Autodesk Fusion 360 part; units mm, degrees
note: some values were not read from the file. Chosen so that the rebuilt part matches the saved one: which bodies a step acts on; a direction; that a step has no effect; which face or edge a step refers to; which pieces of a blend or face edit are solid. Set by a fixed rule: which sketch regions a step uses.
(part 2 of 3)
sketch "Skizze17" plane through (0, 0, -29.4) normal (0, 0, 1) x (1, 0, 0)
  line L0 (185, -2.4) -> (185, 0)
  line L1 (-9.4, 0) -> (-9.4, -2.4)
  line L2 (77.8, 90) -> (97.8, 90)
  line L3 (97.8, 90) -> (97.8, 105)
  line L4 (97.8, 105) -> (77.8, 105)
  line L5 (77.8, 105) -> (77.8, 90)
  circle A0 centre (87.8, 99) radius 2.05
  line L6 (185, -2.4) -> (185, 0)
  line L7 (185, 0) -> (185, 90)
  line L8 (10.6, 105) -> (10.6, 90)
  line L9 (30.6, 90) -> (30.6, 105)
  circle A1 centre (20.6, 99) radius 2.05
  line L10 (10.6, 90) -> (30.6, 90)
  line L11 (30.6, 105) -> (10.6, 105)
  line L12 (185, 0) -> (-9.4, 0)
  line L13 (-9.4, -2.4) -> (185, -2.4)
  dimension "d286" = 20
  dimension "d290" = 4.1
  dimension "d291" = 10
  dimension "d693" = 20
  dimension "d694" = 4.1
  dimension "d695" = 10
  dimension "d701" = 20
  dimension "d703" = 97.2
  dimension "d704" = 99.3749
  dimension "d705" = 15
  dimension "d710" = 6
  constraint horizontal L2
  constraint vertical L3
  constraint horizontal L4
  constraint vertical L5
  constraint horizontal L10
  constraint vertical L9
  constraint horizontal L11
  constraint vertical L8
  constraint horizontal L4.end L9.end
  constraint horizontal A0.centre A1.centre
  measures "d286" distance of L2.start L2.end
  measures "d290" diameter of A0
  measures "d291" distance of L3 A0.centre
  measures "d693" distance of L8.end L9.start
  measures "d694" diameter of A1
  measures "d695" distance of A1.centre L9
  measures "d701" distance of L1.start L8
  measures "d703" distance of L1 A0.centre
  measures "d705" distance of L10 L11
  measures "d710" distance of A1.centre L11
extrude "Extrusion27" add sketch "Skizze17" along normal blind 2.4 from surface at -130.8 contours L2 L3 L4 L5 | L8 L9 L10 L11 bodies 5
sketch "Skizze18" plane through (-9.4, 0, 0) normal (-1, 0, 0) x (0, 0, 1)
  line L0 (8.8, 0) -> (8.8, 81.8)
  line L1 (-120.2, 90) -> (-120.2, 105)
  line L2 (-120.2, 105) -> (-140.2, 105)
  line L3 (-140.2, 105) -> (-140.2, 90)
  circle A0 centre (-130.2, 99) radius 2.05
  line L4 (-29.4, -2.4) -> (-29.4, 0)
  line L5 (-160.2, -2.4) -> (-29.4, -2.4)
  line L6 (-140.2, 90) -> (-120.2, 90)
  line L7 (-49.4, 105) -> (-69.4, 105)
  line L8 (-69.4, 90) -> (-49.4, 90)
  line L9 (-69.4, 105) -> (-69.4, 90)
  line L10 (-49.4, 90) -> (-49.4, 105)
  circle A1 centre (-59.4, 99) radius 2.05
  line L11 (-29.4, 0) -> (-29.4, 90)
  line L12 (-160.2, 90) -> (-29.4, 90)
  line L13 (-29.4, 90) -> (-160.2, 90)
  line L14 (-160.2, 0) -> (-160.2, -2.4)
  line L15 (-29.4, 0) -> (-160.2, 0)
  line L16 (-160.2, 0) -> (-29.4, 0)
  line L17 (-29.4, 0) -> (-29.4, 90)
  line L18 (-160.2, 90) -> (-160.2, 0)
  point P0 (-160.2, 90)
  dimension "d298" = 20
  dimension "d299" = 15
  dimension "d300" = 4.1
  dimension "d301" = 10
  dimension "d687" = 20
  dimension "d688" = 15
  dimension "d689" = 4.1
  dimension "d690" = 10
  dimension "d692" = 20
  dimension "d707" = 6
  dimension "d708" = 6
  dimension "d709" = 20
  constraint vertical L1
  constraint horizontal L2
  constraint vertical L3
  constraint coincident L1 L6.end
  constraint perpendicular L1 L6
  constraint vertical L10
  constraint horizontal L7
  constraint vertical L9
  constraint coincident L8.end L10
  constraint perpendicular L8 L10
  constraint coincident L3.end L12
  constraint coincident L8.start L12
  measures "d298" distance of L3.end L1.start
  measures "d299" distance of L3.end L2.end
  measures "d300" diameter of A0
  measures "d301" distance of L1 A0.centre
  measures "d687" distance of L8.end L8.start
  measures "d688" distance of L8.start L7.end
  measures "d689" diameter of A1
  measures "d690" distance of A1.centre L10
  measures "d692" distance of L10 L11
  measures "d707" distance of A1.centre L7
  measures "d708" distance of L2 A0.centre
  measures "d709" distance of L3 P0
extrude "Extrusion28" add sketch "Skizze18" against normal up to surface (2.4 mm away) contours L1 L2 L3 L6 L12 L13 | L7 L8 L9 L10 L12 L13 bodies 5
chamfer "Fase10" distance 6 distance2 7 4 edges at (97.8, 105, -159) (30.6, 105, -159) (-8.2, 105, -120.2) (-8.2, 105, -49.4) measured on face at (97.8, 95, -158.6) measured on face at (30.6, 95, -158.6) measured on face at (-8.6, 105, -126.8667) measured on face at (-7.8, 105, -56.0667) on bodies 5
chamfer "Fase11" distance 7 distance2 6 4 edges at (-8.2, 105, -69.4) (-8.2, 105, -140.2) (10.6, 105, -159) (77.8, 105, -159) measured on face at (-8.6, 100, -69.4) measured on face at (-8.6, 100, -140.2) measured on face at (14.9333, 105, -159.4) measured on face at (86.4667, 105, -158.6) on bodies 5
sketch "Skizze11" plane through (0, 0, 0) normal (0, 1, 0) x (1, 0, 0)
  line L0 (142.6, 34.4) -> (22.6, 34.4)
  line L1 (22.6, 34.4) -> (22.6, 154.4)
  line L2 (22.6, 154.4) -> (142.6, 154.4)
  line L3 (142.6, 154.4) -> (142.6, 34.4)
  circle A0 centre (82.6, 94.4) radius 57.5
  circle A1 centre (29.6, 147.4) radius 2.5
  circle A2 centre (29.6, 41.4) radius 2.5
  circle A3 centre (135.6, 41.4) radius 2.5
  circle A4 centre (135.6, 147.4) radius 2.5
  line L4 (185, 29.4) -> (185, 160.2)
  circle A5 centre (29.6, 147.4) radius 1.375
  circle A6 centre (135.6, 147.4) radius 1.375
  circle A7 centre (135.6, 41.4) radius 1.375
  circle A8 centre (29.6, 41.4) radius 1.375
  line L5 (22.6, 146.4) -> (142.6, 146.4)
  line L6 (142.6, 146.4) -> (142.6, 142.4)
  line L7 (142.6, 142.4) -> (22.6, 142.4)
  line L8 (22.6, 142.4) -> (22.6, 146.4)
  line L9 (142.6, 140.4) -> (22.6, 140.4)
  line L10 (22.6, 140.4) -> (22.6, 136.4)
  line L11 (22.6, 136.4) -> (142.6, 136.4)
  line L12 (142.6, 136.4) -> (142.6, 140.4)
  line L13 (22.6, 134.4) -> (142.6, 134.4)
  line L14 (142.6, 134.4) -> (142.6, 130.4)
  line L15 (142.6, 130.4) -> (22.6, 130.4)
  line L16 (22.6, 130.4) -> (22.6, 134.4)
  line L17 (142.6, 128.4) -> (22.6, 128.4)
  line L18 (22.6, 128.4) -> (22.6, 124.4)
  line L19 (22.6, 124.4) -> (142.6, 124.4)
  line L20 (142.6, 124.4) -> (142.6, 128.4)
  line L21 (22.6, 122.4) -> (142.6, 122.4)
  line L22 (142.6, 122.4) -> (142.6, 118.4)
  line L23 (142.6, 118.4) -> (22.6, 118.4)
  line L24 (22.6, 118.4) -> (22.6, 122.4)
  line L25 (142.6, 97.4944) -> (142.6, 116.4)
  line L26 (142.6, 116.4) -> (22.6, 116.4)
  line L27 (22.6, 116.4) -> (22.6, 94.4)
  line L28 (142.6, 112.4) -> (22.6, 112.4)
  line L29 (22.6, 112.4) -> (22.6, 110.4)
  line L30 (22.6, 110.4) -> (142.6, 110.4)
  line L31 (142.6, 110.4) -> (142.6, 112.4)
  line L32 (22.6, 106.4) -> (142.6, 106.4)
  line L33 (142.6, 106.4) -> (142.6, 104.4)
  line L34 (142.6, 104.4) -> (22.6, 104.4)
  line L35 (22.6, 104.4) -> (22.6, 106.4)
  line L36 (22.6, 100.4) -> (142.6, 100.4)
  line L37 (142.6, 100.4) -> (142.6, 98.4)
  line L38 (142.6, 98.4) -> (22.6, 98.4)
  line L39 (22.6, 98.4) -> (22.6, 100.4)
  line L40 (142.6, 92.4) -> (22.6, 92.4)
  line L41 (22.6, 92.4) -> (22.6, 94.4)
  line L42 (22.6, 94.4) -> (142.6, 94.4)
  line L43 (142.6, 94.4) -> (142.6, 92.4)
  line L44 (22.6, 88.4) -> (142.6, 88.4)
  line L45 (142.6, 88.4) -> (142.6, 86.4)
  line L46 (142.6, 86.4) -> (22.6, 86.4)
  line L47 (22.6, 86.4) -> (22.6, 88.4)
  line L48 (22.6, 82.4) -> (142.6, 82.4)
  line L49 (142.6, 82.4) -> (142.6, 80.4)
  line L50 (142.6, 80.4) -> (22.6, 80.4)
  line L51 (22.6, 80.4) -> (22.6, 82.4)
  line L52 (142.6, 76.4) -> (22.6, 76.4)
  line L53 (22.6, 76.4) -> (22.6, 74.4)
  line L54 (22.6, 74.4) -> (142.6, 74.4)
  line L55 (142.6, 74.4) -> (142.6, 76.4)
  line L56 (22.6, 70.4) -> (142.6, 70.4)
  line L57 (142.6, 70.4) -> (142.6, 68.4)
  line L58 (142.6, 68.4) -> (22.6, 68.4)
  line L59 (22.6, 68.4) -> (22.6, 70.4)
  line L60 (142.6, 64.4) -> (22.6, 64.4)
  line L61 (22.6, 64.4) -> (22.6, 62.4)
  line L62 (22.6, 62.4) -> (142.6, 62.4)
  line L63 (142.6, 62.4) -> (142.6, 64.4)
  line L64 (22.6, 58.4) -> (142.6, 58.4)
  line L65 (142.6, 58.4) -> (142.6, 56.4)
  line L66 (142.6, 56.4) -> (22.6, 56.4)
  line L67 (22.6, 56.4) -> (22.6, 58.4)
  line L68 (142.6, 50.4) -> (22.6, 50.4)
  line L69 (22.6, 50.4) -> (22.6, 52.4)
  line L70 (22.6, 52.4) -> (142.6, 52.4)
  line L71 (142.6, 52.4) -> (142.6, 50.4)
  line L72 (22.6, 46.4) -> (142.6, 46.4)
  line L73 (142.6, 46.4) -> (142.6, 44.4)
  line L74 (142.6, 44.4) -> (22.6, 44.4)
  line L75 (22.6, 44.4) -> (22.6, 46.4)
  line L76 (142.6, 40.4) -> (22.6, 40.4)
  line L77 (22.6, 40.4) -> (22.6, 37.4)
  line L78 (142.6, 37.4) -> (142.6, 40.4)
  line L79 (51.6, 154.4) -> (53.6, 154.4)
  line L80 (53.6, 154.4) -> (53.6, 34.4)
  line L81 (53.6, 34.4) -> (51.6, 34.4)
  line L82 (51.6, 34.4) -> (51.6, 154.4)
  line L83 (80.6, 154.4) -> (84.6, 154.4)
  line L84 (84.6, 154.4) -> (84.6, 34.4)
  line L85 (84.6, 34.4) -> (80.6, 34.4)
  line L86 (80.6, 34.4) -> (80.6, 154.4)
  line L87 (111.6, 154.4) -> (113.6, 154.4)
  line L88 (113.6, 154.4) -> (113.6, 34.4)
  line L89 (113.6, 34.4) -> (111.6, 34.4)
  line L90 (111.6, 34.4) -> (111.6, 154.4)
  line L91 (182.6, 31.8) -> (-7, 31.8)
  line L92 (-7, 157.8) -> (182.6, 157.8)
  line L93 (-7, 31.8) -> (-7, 157.8)
  line L94 (182.6, 157.8) -> (182.6, 31.8)
  line L95 (-9.4, 120.2) -> (-9.4, 69.4)
  line L96 (13, 156.8) -> (160, 156.8)
  line L97 (-9.4, 160.2) -> (-9.4, 140.2)
  line L98 (-9.4, 49.4) -> (-9.4, 29.4)
  line L99 (-9.4, 29.4) -> (185, 29.4)
  dimension "d208" = 120
  dimension "d209" = 120
  dimension "d213" = 115
  dimension "d214" = 60
  dimension "d215" = 60
  dimension "d216" = 5
  dimension "d217" = 7
  dimension "d218" = 7
  dimension "d219" = 5
  dimension "d220" = 7
  dimension "d221" = 7
  dimension "d222" = 5
  dimension "d223" = 7
  dimension "d224" = 7
  dimension "d225" = 5
  dimension "d226" = 7
  dimension "d227" = 7
  dimension "d334" = 2.75
  dimension "d335" = 2.75
  dimension "d336" = 2.75
  dimension "d337" = 2.75
  dimension "d338" = 8
  dimension "d339" = 4
  dimension "d340" = 2
  dimension "d341" = 4
  dimension "d342" = 2
  dimension "d343" = 4
  dimension "d344" = 2
  dimension "d345" = 4
  dimension "d346" = 2
  dimension "d347" = 4
  dimension "d349" = 2
  dimension "d350" = 4
  dimension "d351" = 2
  dimension "d352" = 4
  dimension "d353" = 2
  dimension "d354" = 4
  dimension "d355" = 2
  dimension "d356" = 4
  dimension "d357" = 2
  dimension "d358" = 4
  dimension "d359" = 2
  dimension "d360" = 4
  dimension "d361" = 2
  dimension "d362" = 4
  dimension "d363" = 2
  dimension "d364" = 4
  dimension "d365" = 2
  dimension "d366" = 4
  dimension "d367" = 2
  dimension "d368" = 4
  dimension "d369" = 2
  dimension "d370" = 4
  dimension "d371" = 2
  dimension "d372" = 4
  dimension "d373" = 2
  dimension "d374" = 4
  dimension "d376" = 2
  dimension "d377" = 4
  dimension "d378" = 2
  dimension "d379" = 2
  dimension "d380" = 29
  dimension "d381" = 29
  dimension "d386" = 1.1639
  dimension "d388" = 45.1997
  dimension "d678" = 40
  dimension "d712" = 2.4
  constraint horizontal L0
  constraint vertical L1
  constraint horizontal L2
  constraint vertical L3
  constraint concentric A1 A5
  constraint concentric A4 A6
  constraint concentric A3 A7
  constraint concentric A2 A8
  constraint horizontal L5
  constraint vertical L6
  constraint horizontal L7
  constraint vertical L8
  constraint coincident L3 L6.end
  constraint coincident L1 L5.start
  constraint horizontal L9
  constraint vertical L10
  constraint horizontal L11
  constraint vertical L12
  constraint coincident L1 L10.end
  constraint coincident L3 L9.start
  constraint horizontal L13
  constraint vertical L14
  constraint horizontal L15
  constraint vertical L16
  constraint coincident L3 L14.end
  constraint coincident L1 L13.start
  constraint horizontal L17
  constraint vertical L18
  constraint horizontal L19
  constraint vertical L20
  constraint coincident L1 L18.end
  constraint coincident L3 L17.start
  constraint horizontal L21
  constraint vertical L22
  constraint horizontal L23
  constraint vertical L24
  constraint coincident L3 L22.end
  constraint coincident L1 L21.start
  constraint vertical L25
  constraint horizontal L26
  constraint vertical L27
  constraint coincident L3 L25.end
  constraint midpoint L1 L27.end
  constraint horizontal L28
  constraint vertical L29
  constraint horizontal L30
  constraint vertical L31
  constraint coincident L1 L29.end
  constraint coincident L3 L28.start
  constraint horizontal L32
  constraint vertical L33
  constraint horizontal L34
  constraint vertical L35
  constraint coincident L3 L33.end
  constraint coincident L1 L32.start
  constraint horizontal L36
  constraint vertical L37
  constraint horizontal L38
  constraint vertical L39
  constraint coincident L3 L37.end
  constraint coincident L1 L36.start
  constraint horizontal L40
  constraint vertical L41
  constraint horizontal L42
  constraint vertical L43
  constraint coincident L3 L40.start
  constraint horizontal L44
  constraint vertical L45
  constraint horizontal L46
  constraint vertical L47
  constraint coincident L3 L45.end
  constraint coincident L1 L44.start
  constraint horizontal L48
  constraint vertical L49
  constraint horizontal L50
  constraint vertical L51
  constraint coincident L3 L49.end
  constraint coincident L1 L48.start
  constraint horizontal L52
  constraint vertical L53
  constraint horizontal L54
  constraint vertical L55
  constraint coincident L1 L53.end
  constraint coincident L3 L52.start
  constraint horizontal L56
  constraint vertical L57
  constraint horizontal L58
  constraint vertical L59
  constraint coincident L3 L57.end
  constraint coincident L1 L56.start
  constraint horizontal L60
  constraint vertical L61
  constraint horizontal L62
  constraint vertical L63
  constraint coincident L1 L61.end
  constraint coincident L3 L60.start
  constraint horizontal L64
  constraint vertical L65
  constraint horizontal L66
  constraint vertical L67
  constraint coincident L3 L65.end
  constraint coincident L1 L64.start
  constraint horizontal L68
  constraint vertical L69
  constraint horizontal L70
  constraint vertical L71
  constraint coincident L1 L69.end
  constraint coincident L3 L68.start
  constraint horizontal L72
  constraint vertical L73
  constraint horizontal L74
  constraint vertical L75
  constraint coincident L3 L73.end
  constraint coincident L1 L72.start
  constraint horizontal L76
  constraint vertical L77
  constraint vertical L78
  constraint coincident L1 L77.end
  constraint coincident L3 L76.start
  constraint horizontal L79
  constraint vertical L80
  constraint horizontal L81
  constraint vertical L82
  constraint coincident L0 L80.end
  constraint coincident L2 L79.start
  constraint horizontal L83
  constraint vertical L84
  constraint horizontal L85
  constraint vertical L86
  constraint coincident L0 L84.end
  constraint coincident L2 L83.start
  constraint horizontal L87
  constraint vertical L88
  constraint horizontal L89
  constraint vertical L90
  constraint coincident L0 L88.end
  constraint coincident L2 L87.start
  constraint coincident L1 L40.end
  measures "d208" distance of L0.start L0.end
  measures "d209" distance of L0.start L2.end
  measures "d213" diameter of A0
  measures "d214" distance of L3 A0.centre
  measures "d215" distance of L0 A0.centre
  measures "d216" diameter of A1
  measures "d217" distance of L1 A1.centre
  measures "d218" distance of L2 A1.centre
  measures "d219" diameter of A2
  measures "d220" distance of L0 A2.centre
  measures "d221" distance of L1 A2.centre
  measures "d222" diameter of A3
  measures "d223" distance of L0 A3.centre
  measures "d224" distance of L3 A3.centre
  measures "d225" diameter of A4
  measures "d226" distance of L3 A4.centre
  measures "d227" distance of L2 A4.centre
  measures "d334" diameter of A5
  measures "d335" diameter of A6
  measures "d336" diameter of A7
  measures "d337" diameter of A8
  measures "d338" distance of L2 L5
  measures "d339" distance of L5 L7
  measures "d340" distance of L7 L9
  measures "d341" distance of L9 L11
  measures "d342" distance of L11 L13
  measures "d343" distance of L13 L15
  measures "d344" distance of L15 L17
  measures "d345" distance of L17 L19
  measures "d346" distance of L19 L21
  measures "d347" distance of L21 L23
  measures "d349" distance of L23 L26
  measures "d350" distance of L26 L28
  measures "d351" distance of L28 L30
  measures "d352" distance of L30 L32
  measures "d353" distance of L32 L34
  measures "d354" distance of L34 L36
  measures "d355" distance of L36 L38
  measures "d356" distance of L38 L42
  measures "d357" distance of L40.start L42
  measures "d358" distance of L40 L44
  measures "d359" distance of L44 L46
  measures "d360" distance of L46 L48
  measures "d361" distance of L48 L50
  measures "d362" distance of L50 L52
  measures "d363" distance of L52 L54
  measures "d364" distance of L54 L56
  measures "d365" distance of L56 L58
  measures "d366" distance of L58 L60
  measures "d367" distance of L60 L62
  measures "d368" distance of L62 L64
  measures "d369" distance of L64 L66
  measures "d370" distance of L66 L70
  measures "d371" distance of L68 L70
  measures "d372" distance of L68 L72
  measures "d373" distance of L72 L74
  measures "d374" distance of L74 L76
  measures "d376" horizontal distance of A0.centre L85.end
  measures "d377" distance of L84 L86
  measures "d378" distance of L88 L90
  measures "d379" distance of L80 L82
  measures "d380" distance of L1 L82
  measures "d381" distance of L3 L88
  measures "d678" distance of L0.start L94
  measures "d712" distance of L2 L96
sketch "Skizze19" plane through (0, 90, 0) normal (0, 1, 0) x (-1, 0, 0)
  line L0 (9.4, -160.2) -> (-185, -160.2)
  line L1 (-185, -160.2) -> (-185, -29.4)
  line L2 (-185, -29.4) -> (9.4, -29.4)
  line L3 (9.4, -29.4) -> (9.4, -160.2)
  line L4 (9.4, -29.4) -> (9.4, -160.2)
  line L5 (9.4, -160.2) -> (-185, -160.2)
  line L6 (-185, -29.4) -> (9.4, -29.4)
  line L7 (7, -157.8) -> (-182.6, -157.8)
  line L8 (-182.6, -157.8) -> (-182.6, -31.8)
  line L9 (-182.6, -31.8) -> (7, -31.8)
  line L10 (7, -31.8) -> (7, -157.8)
  line L11 (7, -157.8) -> (-182.6, -157.8)
  line L12 (7, -31.8) -> (7, -157.8)
  line L13 (-182.6, -31.8) -> (7, -31.8)
  line L14 (9.4, -140.2) -> (7, -140.2)
  line L15 (7, -140.2) -> (7, -120.2)
  line L16 (9.4, -120.2) -> (9.4, -140.2)
  line L17 (9.4, -69.4) -> (7, -69.4)
  line L18 (7, -69.4) -> (7, -49.4)
  line L19 (9.4, -49.4) -> (9.4, -69.4)
  line L20 (4.6, -34.2) -> (-180.2, -34.2)
  line L21 (-180.2, -34.2) -> (-180.2, -155.4)
  line L22 (-180.2, -155.4) -> (4.6, -155.4)
  line L23 (4.6, -155.4) -> (4.6, -34.2)
  line L24 (-10.6, -157.8) -> (-30.6, -157.8)
  line L25 (-30.6, -157.8) -> (-30.6, -160.2)
  line L26 (-30.6, -160.2) -> (-10.6, -160.2)
  line L27 (-10.6, -160.2) -> (-10.6, -157.8)
  line L28 (-77.8, -160.2) -> (-97.8, -160.2)
  line L29 (-97.8, -160.2) -> (-97.8, -157.8)
  line L30 (-97.8, -157.8) -> (-77.8, -157.8)
  line L31 (-77.8, -157.8) -> (-77.8, -160.2)
  line L32 (9.4, -49.4) -> (7, -49.4)
  line L33 (9.4, -120.2) -> (7, -120.2)
  line L34 (-10.6, -160.2) -> (-10.6, -157.8)
  line L35 (-30.6, -157.8) -> (-30.6, -160.2)
  line L36 (-77.8, -160.2) -> (-77.8, -157.8)
  line L37 (-10.6, -160.2) -> (-9.6, -160.2)
  line L38 (-9.6, -160.2) -> (-9.6, -157.8)
  line L39 (-9.6, -157.8) -> (-10.6, -157.8)
  line L40 (-10.6, -157.8) -> (-10.6, -160.2)
  line L41 (-30.6, -160.2) -> (-31.6, -160.2)
  line L42 (-31.6, -160.2) -> (-31.6, -157.8)
  line L43 (-31.6, -157.8) -> (-30.6, -157.8)
  line L44 (-30.6, -157.8) -> (-30.6, -160.2)
  line L45 (7, -140.2) -> (9.4, -140.2)
  line L46 (9.4, -140.2) -> (9.4, -141.2)
  line L47 (9.4, -141.2) -> (7, -141.2)
  line L48 (7, -141.2) -> (7, -140.2)
  line L49 (7, -120.2) -> (9.4, -120.2)
  line L50 (9.4, -120.2) -> (9.4, -119.2)
  line L51 (9.4, -119.2) -> (7, -119.2)
  line L52 (7, -119.2) -> (7, -120.2)
  line L53 (9.4, -49.4) -> (7, -49.4)
  line L54 (7, -49.4) -> (7, -48.4)
  line L55 (7, -48.4) -> (9.4, -48.4)
  line L56 (9.4, -48.4) -> (9.4, -49.4)
  line L57 (7, -69.4) -> (9.4, -69.4)
  line L58 (9.4, -69.4) -> (9.4, -70.4)
  line L59 (9.4, -70.4) -> (7, -70.4)
  line L60 (7, -70.4) -> (7, -69.4)
  line L61 (-77.8, -160.2) -> (-76.8, -160.2)
  line L62 (-76.8, -160.2) -> (-76.8, -157.8)
  line L63 (-76.8, -157.8) -> (-77.8, -157.8)
  line L64 (-77.8, -157.8) -> (-77.8, -160.2)
  line L65 (-97.8, -160.2) -> (-98.8, -160.2)
  line L66 (-98.8, -160.2) -> (-98.8, -157.8)
  line L67 (-98.8, -157.8) -> (-97.8, -157.8)
  line L68 (-97.8, -157.8) -> (-97.8, -160.2)
  point P0 (9.4, -130.2)
  point P1 (9.4, -140.2)
  point P2 (9.4, -69.4)
  point P3 (9.4, -59.4)
  point P4 (-10.6, -29.4)
  point P5 (-20.6, -29.4)
  point P6 (-77.8, -29.4)
  point P7 (-87.8, -29.4)
  point P8 (-145, -29.4)
  point P9 (-155, -29.4)
  point P10 (9.4, -120.2)
  point P11 (9.4, -49.4)
  point P12 (-77.8, -157.8)
  point P13 (-77.8, -160.2)
  point P14 (-97.8, -160.2)
  dimension "d713" = 2.4
  dimension "d714" = 2.4
  dimension "d715" = 2.4
  dimension "d716" = 2.4
  dimension "d758" = 1
  dimension "d759" = 1
  dimension "d760" = 1
  dimension "d761" = 1
  dimension "d762" = 1
  dimension "d763" = 1
  dimension "d764" = 1
  dimension "d765" = 1
  constraint horizontal L0
  constraint vertical L1
  constraint horizontal L2
  constraint vertical L3
  constraint coincident L0.start L4
  constraint coincident L0.start L5
  constraint coincident L2.end L6
  constraint coincident L1 L2.start
  constraint horizontal L7
  constraint vertical L8
  constraint horizontal L9
  constraint vertical L10
  constraint coincident L7.start L11
  constraint coincident L7.start L12
  constraint coincident L9.end L13
  constraint coincident L8 L9.start
  constraint horizontal L14
  constraint vertical L15
  constraint vertical L16
  constraint coincident L10 L15.end
  constraint coincident L3 P1
  constraint horizontal L17
  constraint vertical L18
  constraint vertical L19
  constraint coincident L12 L18.end
  constraint coincident L3 P2
  constraint coincident L14 P1
  constraint coincident L17 P2
  constraint horizontal L20
  constraint vertical L21
  constraint horizontal L22
  constraint vertical L23
  constraint horizontal L24
  constraint vertical L25
  constraint horizontal L26
  constraint vertical L27
  constraint coincident L0 L25.end
  constraint coincident L7 L24.start
  constraint horizontal L28
  constraint vertical L29
  constraint horizontal L30
  constraint vertical L31
  constraint coincident L7 L29.end
  constraint coincident L0 P13
  constraint coincident L10 L18.end
  constraint perpendicular L10 L32
  constraint perpendicular L10 L33
  constraint coincident L26.end L34
  constraint coincident L25.end L35
  constraint coincident P13 L36
  constraint horizontal L37
  constraint vertical L38
  constraint horizontal L39
  constraint vertical L40
  constraint coincident L26.end L27.start
  constraint horizontal L41
  constraint vertical L42
  constraint horizontal L43
  constraint vertical L44
  constraint coincident L25.end L26.start
  constraint horizontal L45
  constraint vertical L46
  constraint horizontal L47
  constraint vertical L48
  constraint horizontal L49
  constraint vertical L50
  constraint horizontal L51
  constraint vertical L52
  constraint coincident P10 L16.start
  constraint coincident L32 P11
  constraint horizontal L53
  constraint vertical L54
  constraint horizontal L55
  constraint vertical L56
  constraint coincident P11 L19.start
  constraint horizontal L57
  constraint vertical L58
  constraint horizontal L59
  constraint vertical L60
  constraint horizontal L61
  constraint vertical L62
  constraint horizontal L63
  constraint vertical L64
  constraint coincident P13 L28.start
  constraint horizontal L65
  constraint vertical L66
  constraint horizontal L67
  constraint vertical L68
  measures "d713" distance of L7 L22
  measures "d714" distance of L10 L23
  measures "d715" distance of L9 L20
  measures "d716" distance of L8 L21
  measures "d758" distance of L26.end L37.end
  measures "d759" distance of L25.end L41.end
  measures "d760" distance of L14.end L47.end
  measures "d761" distance of L15.end L51.end
  measures "d762" distance of P11 L55.end
  measures "d763" distance of L17.end L59.end
  measures "d764" distance of P13 L61.end
  measures "d765" distance of P14 L65.end
extrude "Extrusion29" add sketch "Skizze19" along normal blind 2 from surface at 5 separate body contours L0 L3 L4 L5 L7 L10 L11 L12 L38 L47 | L0 L5 L7 L11 L27 L34 L37 L38 L39 L40 | L3 L4 L10 L12 L14 L45 L46 L47 L48 | L0 L5 L7 L11 L24 L25 L26 L27 L34 L35 L40 L44 | L7 L8 L9 L10 L11 L12 L13 L15 L18 L24 L30 L39 L43 L48 L52 L54 L60 L63 L67 | L3 L4 L10 L12 L14 L15 L16 L33 L45 L49 | L0 L5 L7 L11 L25 L35 L41 L42 L43 L44 | L3 L4 L10 L12 L33 L49 L50 L51 L52 | L0 L5 L7 L11 L42 L62 | L3 L4 L10 L12 L51 L59 | L0 L5 L7 L11 L31 L36 L61 L62 L63 L64 | L3 L4 L10 L12 L17 L57 L58 L59 L60 | L0 L5 L7 L11 L28 L29 L30 L31 L36 L64 L68 | L3 L4 L10 L12 L17 L18 L19 L32 L53 L57 | L0 L5 L7 L11 L29 L65 L66 L67 L68 | L3 L4 L10 L12 L32 L53 L54 L55 L56 | L0 L1 L2 L3 L4 L5 L6 L7 L8 L9 L10 L11 L12 L13 L55 L66 | L20 L21 L22 L23 makes body 8
extrude "Extrusion30" add sketch "Skizze19" against normal blind 2 from surface at 5 separate body contours L7 L8 L9 L10 L11 L12 L13 L15 L18 L24 L30 L39 L43 L48 L52 L54 L60 L63 L67 makes body 9
extrude "Extrusion59" cut sketch "Skizze9" against normal blind 10 from surface at 97 contours A8 | A10 | A12 | A15 bodies 8 9
fillet "Abrundung2" radius 1 4 edges at (87.8, 93, -31.8) (-7, 93, -94.8) (182.6, 93, -94.8) (87.8, 93, -157.8) on bodies 9
extrude "Extrusion31" add sketch "Skizze11" against normal blind 7 from surface at 95 contours A3 A7 L76 | A3 A7 L76 | A2 A8 L76 | A2 A8 L76 | A4 A6 L5 | A4 A6 L5 | A1 A5 L5 | A1 A5 L5 bodies 8
combine "Kombinieren6" operation add target body 8 tool bodies 9
extrude "Extrusion32" cut sketch "Skizze11" against normal up to surface (2 mm away) from surface at 97 contours A0 L74 L76 L84 | A0 L72 L88 | A0 L68 L72 L88 | A0 L74 L76 L86 | L68 L72 L84 L90 | A0 L66 L70 L88 | L68 L72 L80 L86 | L66 L70 L84 L90 | A0 L72 L82 | A0 L62 L64 L88 | A0 L68 L72 L82 | L66 L70 L80 L86 | L62 L64 L84 L90 | A0 L58 L60 L88 | A0 L66 L70 L82 | L62 L64 L80 L86 | L58 L60 L84 L90 | A0 L54 L56 L88 | A0 L62 L64 L82 | L58 L60 L80 L86 | L54 L56 L84 L90 | A0 L50 L52 L88 | A0 L58 L60 L82 | L54 L56 L80 L86 | L50 L52 L84 L90 | A0 L46 L48 L88 | A0 L54 L56 L82 | L50 L52 L80 L86 | L46 L48 L84 L90 | A0 L40 L44 L88 | A0 L50 L52 L82 | L46 L48 L80 L86 | L40 L44 L84 L90 | A0 L38 L42 L88 | A0 L46 L48 L82 | L40 L44 L80 L86 | L38 L42 L84 L90 | A0 L34 L36 L88 | A0 L40 L44 L82 | L38 L42 L80 L86 | L34 L36 L84 L90 | A0 L30 L32 L88 | A0 L38 L42 L82 | L34 L36 L80 L86 | L30 L32 L84 L90 | A0 L26 L28 L88 | A0 L34 L36 L82 | L30 L32 L80 L86 | L26 L28 L84 L90 | A0 L21 L23 L88 | A0 L30 L32 L82 | L26 L28 L80 L86 | L21 L23 L84 L90 | A0 L17 L19 L88 | A0 L26 L28 L82 | L21 L23 L80 L86 | L17 L19 L84 L90 | A0 L13 L15 L88 | A0 L21 L23 L82 | L17 L19 L80 L86 | L13 L15 L84 L90 | A0 L9 L11 L88 | A0 L17 L19 L82 | L13 L15 L80 L86 | L9 L11 L84 L90 | A0 L13 L15 L82 | L9 L11 L80 L86 | A0 L5 L7 L84 L90 | A0 L9 L11 L82 | A0 L5 L7 L80 L86 bodies 8
extrude "Extrusion65" cut sketch "Skizze19" along normal up to surface (7 mm away) and the other way blind 0 contours L0 L5 L7 L11 L27 L34 L37 L38 L39 L40 | L3 L4 L10 L12 L14 L45 L46 L47 L48 | L0 L5 L7 L11 L24 L25 L26 L27 L34 L35 L40 L44 | L3 L4 L10 L12 L14 L15 L16 L33 L45 L49 | L0 L5 L7 L11 L25 L35 L41 L42 L43 L44 | L3 L4 L10 L12 L33 L49 L50 L51 L52 | L0 L5 L7 L11 L31 L36 L61 L62 L63 L64 | L3 L4 L10 L12 L17 L57 L58 L59 L60 | L0 L5 L7 L11 L28 L29 L30 L31 L36 L64 L68 | L3 L4 L10 L12 L17 L18 L19 L32 L53 L57 | L0 L5 L7 L11 L29 L65 L66 L67 L68 | L3 L4 L10 L12 L32 L53 L54 L55 L56 bodies 8
extrude "Extrusion23" add sketch "Skizze11" against normal blind 15 from surface at 90 separate body contours L0 L3 A3 L76 L78 L88 | L0 L76 L88 L89 L90 | L0 A0 L76 L84 L90 | L3 A3 L74 L76 L88 | L74 L76 L88 L90 | L0 A0 L84 L85 L86 | A0 L74 L76 L90 | L3 A0 L72 L73 L74 L88 | A0 L74 L88 L90 | L0 A0 L76 L80 L86 | A0 L74 L90 | L3 A0 L68 L72 | L0 L76 L80 L81 L82 | L3 A0 L68 L70 L71 | L0 L1 A2 L76 L77 L82 | A0 L74 L76 L80 | L74 L76 L80 L82 | L3 A0 L66 L70 | L1 A2 L74 L76 L82 | A0 L74 L80 | A0 L74 L80 L82 | L3 A0 L64 L65 L66 | L1 A0 L72 L74 L75 L82 | L3 A0 L62 L64 | L3 A0 L60 L62 L63 | L1 A0 L68 L72 | L3 A0 L58 L60 | L1 A0 L68 L69 L70 | L3 A0 L56 L57 L58 | L1 A0 L66 L70 | L3 A0 L54 L56 | L1 A0 L64 L66 L67 | L3 A0 L52 L54 L55 | L1 A0 L62 L64 | L3 A0 L50 L52 | L1 A0 L60 L61 L62 | L3 A0 L48 L49 L50 | L1 A0 L58 L60 | L3 A0 L46 L48 | L1 A0 L56 L58 L59 | L3 A0 L44 L45 L46 | L1 A0 L54 L56 | L3 A0 L40 L44 | L1 A0 L52 L53 L54 | L3 A0 L40 L42 L43 | L1 A0 L50 L52 | L3 A0 L25 L38 L42 | L1 A0 L48 L50 L51 | L1 A0 L46 L48 | L3 A0 L25 L36 L37 L38 | L1 A0 L44 L46 L47 | L3 A0 L25 L34 L36 | L1 A0 L40 L44 | L3 A0 L25 L32 L33 L34 | L1 A0 L40 L41 L42 | L3 A0 L25 L30 L32 | L1 A0 L27 L38 L42 | L3 A0 L25 L28 L30 L31 | L1 A0 L27 L36 L38 L39 | L3 A0 L25 L26 L28 | L1 A0 L27 L34 L36 | L3 A0 L23 L26 | L1 A0 L27 L32 L34 L35 | L3 A0 L21 L22 L23 | L1 A0 L27 L30 L32 | L3 A0 L19 L21 | L1 A0 L27 L28 L29 L30 | L3 A0 L17 L19 L20 | L1 A0 L26 L27 L28 | L3 A0 L15 L17 | L1 A0 L23 L26 | L3 A0 L13 L14 L15 | L1 A0 L21 L23 L24 | L3 A0 L11 L13 | L1 A0 L19 L21 | L3 A0 L9 L11 L12 | L1 A0 L17 L18 L19 | L3 A0 L7 L9 | L1 A0 L15 L17 | L3 A0 A4 L5 L6 L7 L88 | L1 A0 L13 L15 L16 | A0 L5 L88 L90 | L2 L3 A4 L5 L88 | L1 A0 L11 L13 | A0 L5 L90 | L2 L5 L87 L88 L90 | L1 A0 L9 L10 L11 | L2 A0 L5 L84 L90 | L1 A0 L7 L9 | L2 A0 L83 L84 L86 | L1 A0 A1 L5 L7 L8 L82 | A0 L5 L80 | A0 L5 L80 L82 | L2 A0 L5 L80 L86 | L1 L2 A1 L5 L82 | L2 L5 L79 L80 L82 makes body 10
sketch "Skizze28" plane through (0, 90, 0) normal (0, 1, 0) x (-1, 0, 0)
  line L0 (-80.6, -34.4) -> (-84.6, -34.4)
  line L1 (-84.6, -34.4) -> (-84.6, -156.6872)
  line L2 (-84.6, -156.6872) -> (-80.6, -156.6872)
  line L3 (-80.6, -156.6872) -> (-80.6, -34.4)
  line L4 (-53.6, -156.6872) -> (-51.6, -156.6872)
  line L5 (-51.6, -156.6872) -> (-51.6, -34.4)
  line L6 (-51.6, -34.4) -> (-53.6, -34.4)
  line L7 (-53.6, -34.4) -> (-53.6, -156.6872)
  line L8 (-111.6, -34.4) -> (-113.6, -34.4)
  line L9 (-113.6, -34.4) -> (-113.6, -156.6872)
  line L10 (-113.6, -156.6872) -> (-111.6, -156.6872)
  line L11 (-111.6, -156.6872) -> (-111.6, -34.4)
  line L12 (-142.6, -94.4) -> (-22.6, -94.4)
  line L13 (-22.6, -94.4) -> (-22.6, -92.4)
  line L14 (-22.6, -92.4) -> (-142.6, -92.4)
  line L15 (-142.6, -92.4) -> (-142.6, -94.4)
  line L16 (-139.6, -64.4) -> (-22.6, -64.4)
  line L17 (-22.6, -64.4) -> (-22.6, -62.4)
  line L18 (-22.6, -62.4) -> (-139.6, -62.4)
  line L19 (-139.6, -62.4) -> (-139.6, -64.4)
  line L20 (-139.6, -124.4) -> (-22.6, -124.4)
  line L21 (-22.6, -124.4) -> (-22.6, -122.4)
  line L22 (-22.6, -122.4) -> (-139.6, -122.4)
  line L23 (-139.6, -122.4) -> (-139.6, -124.4)
  line L24 (-22.6, -62.4) -> (-142.6, -62.4)
  line L25 (-142.6, -64.4) -> (-22.6, -64.4)
  line L26 (-22.6, -34.4) -> (-25.6, -34.4)
  line L27 (-25.6, -34.4) -> (-25.6, -156.6872)
  line L28 (-25.6, -156.6872) -> (-22.6, -156.6872)
  line L29 (-22.6, -156.6872) -> (-22.6, -34.4)
  line L30 (-22.6, -34.4) -> (-22.6, -154.4)
  line L31 (-116.5619, -156.6872) -> (-60.8294, -156.6872)
  line L32 (-139.6, 11.1172) -> (-142.6, 11.1172)
  line L33 (-142.6, 11.1172) -> (-142.6, -156.6872)
  line L34 (-142.6, -156.6872) -> (-139.6, -156.6872)
  line L35 (-139.6, -156.6872) -> (-139.6, 11.1172)
  line L36 (-142.6, -154.4) -> (-142.6, -34.4)
  line L37 (-51.6, -92.4) -> (-25.1348, -92.4)
  line L38 (-25.1, -94.4) -> (-51.6, -94.4)
  line L39 (-51.6, -122.4) -> (-32.378, -122.4)
  line L40 (-33.5465, -124.4) -> (-51.6, -124.4)
  line L41 (-22.6, -80.4) -> (-139.6, -80.4)
  line L42 (-139.6, -80.4) -> (-139.6, -82.4)
  line L43 (-139.6, -82.4) -> (-22.6, -82.4)
  line L44 (-22.6, -82.4) -> (-22.6, -80.4)
  line L45 (-22.6, -104.4) -> (-139.6, -104.4)
  line L46 (-139.6, -104.4) -> (-139.6, -106.4)
  line L47 (-139.6, -106.4) -> (-22.6, -106.4)
  line L48 (-22.6, -106.4) -> (-22.6, -104.4)
  line L49 (-22.6, -134.4) -> (-139.6, -134.4)
  line L50 (-139.6, -134.4) -> (-139.6, -136.4)
  line L51 (-139.6, -136.4) -> (-22.6, -136.4)
  line L52 (-22.6, -136.4) -> (-22.6, -134.4)
  line L53 (-22.6, -50.4) -> (-139.6, -50.4)
  line L54 (-139.6, -50.4) -> (-139.6, -52.4)
  line L55 (-139.6, -52.4) -> (-22.6, -52.4)
  line L56 (-22.6, -52.4) -> (-22.6, -50.4)
  line L57 (-142.6, -50.4) -> (-22.6, -50.4)
  line L58 (-22.6, -52.4) -> (-142.6, -52.4)
  line L59 (-22.6, -156.6872) -> (-142.6, -156.6872)
  line L60 (-142.6, -156.6872) -> (-142.6, -159.6872)
  line L61 (-142.6, -159.6872) -> (-22.6, -159.6872)
  line L62 (-22.6, -159.6872) -> (-22.6, -156.6872)
  line L63 (-22.6, -34.4) -> (-142.6, -34.4)
  line L64 (-142.6, -34.4) -> (-142.6, -31.4)
  line L65 (-142.6, -31.4) -> (-22.6, -31.4)
  line L66 (-22.6, -31.4) -> (-22.6, -34.4)
  line L67 (-25.6, -50.4) -> (-51.6, -34.4)
  line L68 (-113.6, -34.4) -> (-139.6, -50.4)
  line L69 (-51.6, -156.6872) -> (-25.6, -136.4)
  line L70 (-113.6, -156.6872) -> (-139.6, -136.4)
  point P0 (-80.6, -34.4)
  point P1 (-84.6, -34.4)
  point P2 (-51.6, -34.4)
  point P3 (-53.6, -34.4)
  point P4 (-111.6, -34.4)
  point P5 (-113.6, -34.4)
  point P6 (-22.6, -154.4)
  point P7 (-22.6, -80.4)
  point P8 (-22.6, -82.4)
  point P9 (-22.6, -134.4)
  point P10 (-22.6, -136.4)
  point P11 (-22.6, -104.4)
  point P12 (-22.6, -106.4)
  point P13 (-22.6, -34.4)
  dimension "d630" = 3
  dimension "d631" = 3
  dimension "d657" = 3
  dimension "d658" = 3
  constraint horizontal L0
  constraint vertical L1
  constraint horizontal L2
  constraint vertical L3
  constraint horizontal L4
  constraint vertical L5
  constraint horizontal L6
  constraint vertical L7
  constraint horizontal L8
  constraint vertical L9
  constraint horizontal L10
  constraint vertical L11
  constraint horizontal L12
  constraint vertical L13
  constraint horizontal L14
  constraint vertical L15
  constraint horizontal L16
  constraint vertical L17
  constraint horizontal L18
  constraint vertical L19
  constraint horizontal L20
  constraint vertical L21
  constraint horizontal L22
  constraint vertical L23
  constraint horizontal P0 P2
  constraint horizontal P0 P4
  constraint coincident L3 P0
  constraint coincident L1 P1
  constraint coincident L7 P3
  constraint coincident L11 P4
  constraint coincident L9 P5
  constraint coincident L16.end L25
  constraint horizontal L26
  constraint vertical L27
  constraint horizontal L28
  constraint vertical L29
  constraint coincident L28.end L30
  constraint coincident L28.end L31
  constraint coincident L4.end L31
  constraint coincident L2.end L31
  constraint coincident L10.end L31
  constraint horizontal L32
  constraint vertical L33
  constraint horizontal L34
  constraint vertical L35
  constraint coincident L31 L33.end
  constraint coincident L32.end L36
  constraint coincident L17.end L18.start
  constraint coincident L13.end L37
  constraint coincident L12.end L38
  constraint coincident L21.end L39
  constraint coincident L20.end L40
  constraint horizontal L41
  constraint vertical L42
  constraint horizontal L43
  constraint vertical L44
  constraint coincident L35 L42.end
  constraint coincident L29 P7
  constraint horizontal L45
  constraint vertical L46
  constraint horizontal L47
  constraint vertical L48
  constraint coincident L35 L46.end
  constraint coincident L30 P11
  constraint horizontal L49
  constraint vertical L50
  constraint horizontal L51
  constraint vertical L52
  constraint coincident L35 L50.end
  constraint coincident L30 P9
  constraint horizontal L53
  constraint vertical L54
  constraint horizontal L55
  constraint vertical L56
  constraint coincident L35 L54.end
  constraint coincident L30 L53.start
  constraint coincident L53.start L57
  constraint coincident L55.end L58
  constraint coincident L41 P7
  constraint coincident L43 P8
  constraint coincident L49 P9
  constraint coincident L51 P10
  constraint coincident L45 P11
  constraint coincident L47 P12
  constraint horizontal L59
  constraint vertical L60
  constraint horizontal L61
  constraint vertical L62
  constraint horizontal L63
  constraint vertical L64
  constraint horizontal L65
  constraint vertical L66
  constraint coincident L32.end L64
  constraint coincident L27 L67.start
  constraint coincident L53 L67.start
  constraint coincident P5 L8.end
  constraint coincident L27 L69.end
  constraint coincident L51 L69.end
  constraint horizontal L31
  constraint coincident L21.end L29
  constraint coincident L13.end L29
  constraint coincident L33 L60.end
  constraint coincident P2 L63
  constraint coincident L63 P13
  constraint coincident P2 L5.end
  constraint coincident L22.end L35
  constraint coincident L18.end L35
  measures "d630" horizontal distance of L27.end P6
  measures "d631" distance of L33 L35
  measures "d657" distance of L28.end L61.end
  measures "d658" distance of P13 L65.end
extrude "Extrusion55" add sketch "Skizze28" against normal blind 2 from surface at -15 separate body contours L0 L1 L3 L53 L57 L63 | L0 L6 L8 L26 L35 L63 L65 L66 | L3 L7 L53 L55 L57 L58 | L1 L3 L53 L55 L57 L58 | L5 L6 L7 L53 L57 L63 | L1 L11 L53 L55 L57 L58 | L8 L9 L11 L53 L57 L63 | L1 L3 L18 L24 L55 L58 | L5 L7 L53 L55 L57 L58 | L27 L63 L67 | L9 L11 L53 L55 L57 L58 | L35 L63 L68 | L3 L7 L16 L18 L24 L25 | L1 L3 L16 L18 L24 L25 | L5 L7 L18 L24 L55 L58 | L5 L27 L53 L55 L57 L58 | L26 L27 L29 L30 L53 L57 L63 | L27 L29 L30 L53 L55 L56 L57 L58 | L1 L11 L16 L18 L24 L25 | L9 L11 L18 L24 L55 L58 | L9 L35 L53 L54 L55 L57 L58 | L33 L35 L63 L64 L65 | L33 L35 L36 L57 L63 | L33 L35 L36 L54 L57 L58 | L1 L3 L16 L25 L41 | L5 L7 L16 L18 L24 L25 | L18 L24 L27 L29 L30 L55 L58 | L9 L11 L16 L18 L24 L25 | L24 L33 L35 L36 L58 | L3 L7 L41 L43 | L1 L3 L41 L43 | L5 L7 L16 L25 L41 | L5 L16 L18 L24 L25 L27 | L16 L17 L18 L24 L25 L27 L29 L30 | L1 L11 L41 L43 | L9 L11 L16 L25 L41 | L9 L16 L18 L19 L24 L25 L35 | L19 L24 L25 L33 L35 L36 | L1 L3 L14 L43 | L5 L7 L41 L43 | L16 L25 L27 L29 L30 L41 | L9 L11 L41 L43 | L14 L25 L33 L35 L36 L42 | L3 L7 L12 L14 | L1 L3 L12 L14 | L5 L7 L14 L43 | L5 L27 L41 L43 | L27 L29 L30 L41 L43 L44 | L1 L11 L12 L14 | L9 L11 L14 L43 | L9 L35 L41 L42 L43 | L1 L3 L12 L45 | L5 L7 L12 L14 | L14 L27 L29 L30 L37 L43 | L9 L11 L12 L14 | L12 L14 L15 L33 L35 L36 | L3 L7 L45 L47 | L1 L3 L45 L47 | L5 L7 L12 L45 | L5 L12 L14 L27 L37 L38 | L12 L13 L14 L27 L29 L30 L37 L38 | L1 L11 L45 L47 | L9 L11 L12 L45 | L9 L12 L14 L35 | L12 L23 L33 L34 L35 L36 L46 L50 L59 | L1 L3 L22 L47 | L5 L7 L45 L47 | L12 L27 L29 L30 L38 L45 | L9 L11 L45 L47 | L3 L7 L20 L22 | L1 L3 L20 L22 | L5 L7 L22 L47 | L5 L27 L45 L47 | L27 L29 L30 L45 L47 L48 | L1 L11 L20 L22 | L9 L11 L22 L47 | L9 L35 L45 L46 L47 | L2 L4 L10 L28 L31 L34 L59 L60 L61 L62 | L1 L3 L20 L49 | L5 L7 L20 L22 | L22 L27 L29 L30 L47 | L9 L11 L20 L22 | L31 L35 L59 L70 | L3 L7 L49 L51 | L1 L3 L49 L51 | L5 L7 L20 L49 | L5 L20 L22 L27 L39 L40 | L20 L21 L22 L27 L29 L30 | L1 L11 L49 L51 | L9 L11 L20 L49 | L9 L20 L22 L23 L35 | L9 L35 L49 L50 L51 | L1 L2 L3 L31 L51 L59 | L5 L7 L49 L51 | L20 L27 L29 L30 L49 | L9 L11 L49 L51 | L9 L10 L11 L31 L51 L59 | L27 L28 L29 L30 L51 L59 | L4 L5 L7 L51 L59 | L5 L27 L49 L51 | L27 L29 L30 L49 L51 L52 | L27 L59 L69 makes body 11
extrude "Extrusion60" cut sketch "Skizze11" along normal up to surface (2 mm away) from surface at 73 contours A7 L76 | A7 L76 | A8 L76 | A8 L76 | A6 L5 | A6 L5 | A5 L5 | A5 L5 bodies 11
move_body "Verschieben3" bodies 1 2 3 to x (1, 0, 0) y (0, 1, 0) z (0, 0, 1) at (0, 0, 56)
sketch "Skizze21" plane through (0, 28.4, 0) normal (0, 1, 0) x (-1, 0, 0)
  line L0 (-122, 49) -> (7, 49)
  line L1 (7, 49) -> (7, 346)
  line L2 (7, 346) -> (-122, 346)
  line L3 (-122, 346) -> (-122, 49)
  line L4 (7, 187.2) -> (-122, 187.2)
  line L5 (7, 172.2) -> (-3, 172.2)
  line L6 (-3, 172.2) -> (-3, 202.2)
  line L7 (-3, 202.2) -> (7, 202.2)
  line L8 (7, 202.2) -> (7, 172.2)
  line L9 (-122, 172.2) -> (-112, 172.2)
  line L10 (-112, 172.2) -> (-112, 202.2)
  line L11 (-112, 202.2) -> (-122, 202.2)
  line L12 (-122, 202.2) -> (-122, 172.2)
  line L13 (-3, 172.2) -> (7, 172.2)
  line L14 (7, 172.2) -> (7, 162.2)
  line L15 (7, 162.2) -> (-3, 162.2)
  line L16 (-3, 162.2) -> (-3, 172.2)
  line L17 (-122, 172.2) -> (-112, 172.2)
  line L18 (-112, 172.2) -> (-112, 162.2)
  line L19 (-112, 162.2) -> (-122, 162.2)
  line L20 (-122, 162.2) -> (-122, 172.2)
  circle A0 centre (2, 179.7) radius 1.25
  circle A1 centre (-117, 179.7) radius 1.25
  line L21 (-50.5, 172.2) -> (-60.5, 172.2)
  line L22 (-60.5, 172.2) -> (-60.5, 202.2)
  line L23 (-60.5, 202.2) -> (-50.5, 202.2)
  line L24 (-50.5, 202.2) -> (-50.5, 172.2)
  line L25 (-50.5, 172.2) -> (-60.5, 172.2)
  line L26 (-60.5, 172.2) -> (-60.5, 162.2)
  line L27 (-60.5, 162.2) -> (-50.5, 162.2)
  line L28 (-50.5, 162.2) -> (-50.5, 172.2)
  circle A2 centre (-55.5, 179.8) radius 1.25
  line L29 (7, 197.5) -> (-122, 197.5)
  line L30 (-8, 171) -> (-107, 171)
  line L31 (-107, 171) -> (-107, 196)
  line L32 (-107, 196) -> (-8, 196)
  line L33 (-8, 196) -> (-8, 171)
  line L34 (-8, 276) -> (-107, 276)
  line L35 (-107, 276) -> (-107, 301)
  line L36 (-107, 301) -> (-8, 301)
  line L37 (-8, 301) -> (-8, 276)
  line L38 (-8, 136) -> (-107, 136)
  line L39 (-107, 136) -> (-107, 161)
  line L40 (-107, 161) -> (-8, 161)
  line L41 (-8, 161) -> (-8, 136)
  line L42 (-8, 206) -> (-107, 206)
  line L43 (-107, 206) -> (-107, 231)
  line L44 (-107, 231) -> (-8, 231)
  line L45 (-8, 231) -> (-8, 206)
  line L46 (-8, 241) -> (-107, 241)
  line L47 (-107, 241) -> (-107, 266)
  line L48 (-107, 266) -> (-8, 266)
  line L49 (-8, 266) -> (-8, 241)
  line L50 (-8, 101) -> (-107, 101)
  line L51 (-107, 101) -> (-107, 126)
  line L52 (-107, 126) -> (-8, 126)
  line L53 (-8, 126) -> (-8, 101)
  point P0 (7, 187.2)
  dimension "d399" = 30
  dimension "d400" = 10
  dimension "d401" = 15
  dimension "d402" = 30
  dimension "d403" = 10
  dimension "d404" = 15
  dimension "d408" = 10
  dimension "d409" = 10
  dimension "d416" = 2.5
  dimension "d417" = 7.5
  dimension "d418" = 5
  dimension "d419" = 2.5
  dimension "d420" = 5
  dimension "d421" = 7.5
  dimension "d423" = 10
  dimension "d424" = 30
  dimension "d425" = 15
  dimension "d426" = 57.5
  dimension "d427" = 10
  dimension "d428" = 10
  dimension "d429" = 2.5
  dimension "d430" = 7.6
  dimension "d431" = 5
  constraint coincident L3 L4.end
  constraint horizontal L4
  constraint coincident L1 P0
  constraint coincident P0 L4.start
  constraint horizontal L5
  constraint vertical L6
  constraint horizontal L7
  constraint vertical L8
  constraint coincident L1 L5.start
  constraint horizontal L9
  constraint vertical L10
  constraint horizontal L11
  constraint vertical L12
  constraint coincident L3 L9.start
  constraint horizontal L13
  constraint vertical L14
  constraint horizontal L15
  constraint vertical L16
  constraint horizontal L17
  constraint vertical L18
  constraint horizontal L19
  constraint vertical L20
  constraint horizontal L21
  constraint vertical L22
  constraint horizontal L23
  constraint vertical L24
  constraint horizontal L25
  constraint vertical L26
  constraint horizontal L27
  constraint vertical L28
  constraint midpoint L1 L29.start
  constraint midpoint L3 L29.end
  measures "d399" distance of L5.start L7.end
  measures "d400" distance of L5.start L5.end
  measures "d401" distance of L4 L5
  measures "d402" distance of L9.start L11.end
  measures "d403" distance of L9.start L9.end
  measures "d404" distance of L4 L9
  measures "d408" distance of L5.end L15.end
  measures "d409" distance of L9.start L19.end
  measures "d416" diameter of A0
  measures "d417" distance of L13 A0.centre
  measures "d418" distance of L6 A0.centre
  measures "d419" diameter of A1
  measures "d420" distance of L12 A1.centre
  measures "d421" distance of L4 A1.centre
  measures "d423" distance of L21.start L21.end
  measures "d424" distance of L21.start L23.end
  measures "d425" distance of L4 L21
  measures "d426" distance of L8 L24
  measures "d427" distance of L21.start L21.end
  measures "d428" distance of L21.start L27.end
  measures "d429" diameter of A2
  measures "d430" distance of L25 A2.centre
  measures "d431" distance of L22 A2.centre
split "Teilen1" by curves path "Skizze21" along L4 bodies 1 makes body 12 at (41, 26, 333.6667)
extrude "Extrusion33" add sketch "Skizze21" along normal blind 2.4 separate body contours L3 L4 L9 L10 L12 L17 | L1 L4 L5 L6 L8 L13 | L3 L4 L10 L12 L29 | L1 L4 L6 L8 L29 | L3 L10 L11 L12 L29 | L1 L6 L7 L8 L29 | L22 L24 L29 L32 | L22 L23 L24 L29 | L4 L22 L24 L32 | L4 L21 L22 L24 L25 | A0 | A1 | A2 makes body 13 at (-3.6667, 28.4, 182.2) makes body 14 at (115.3333, 28.4, 182.2) makes body 15 at (57.1667, 28.4, 192.2)
extrude "Extrusion34" add sketch "Skizze21" along normal blind 4.8 separate body contours L3 L9 L17 L18 L19 L20 | L1 L5 L13 L14 L15 L16 | L21 L25 L26 L28 L30 | L26 L27 L28 L30 makes body 16 at (-0.3333, 28.4, 165.5333) makes body 17 at (118.6667, 28.4, 168.8667) makes body 18 at (57.1667, 28.4, 168.8667)
extrude "Extrusion35" add sketch "Skizze21" along normal blind 2.4 from surface at 2.4 separate body contours L3 L4 L9 L10 L12 L17 | L1 L4 L5 L6 L8 L13 | L4 L21 L22 L24 L25 | A0 | A1 | A2 makes body 19 at (118.6667, 30.8, 182.2) makes body 20 at (-0.3333, 30.8, 177.2) makes body 21 at (57.1667, 30.8, 182.2)
combine "Kombinieren1" operation add target body 12 tool bodies 13 14 15
combine "Kombinieren3" operation add target body 16 tool bodies 17 19 20 1 18 21
extrude "Extrusion36" cut sketch "Skizze21" along normal through all and the other way through all from surface at -2.4 contours A0 | A1 | A2 bodies 12 16
sketch "Skizze23" plane through (-7, 0, 0) normal (1, 0, 0) x (0, 0, -1)
  circle A0 centre (-261, 51) radius 7.85
  line L0 (-202.2, 28.4) -> (-202.2, 30.8)
  line L1 (-202.2, 30.8) -> (-187.2, 30.8)
  line L2 (-187.2, 30.8) -> (-187.2, 80)
  line L3 (-187.2, 80) -> (-346, 80)
  line L4 (-346, 80) -> (-346, 28.4)
  line L5 (-346, 28.4) -> (-202.2, 28.4)
  line L6 (-202.2, 92.4) -> (-172.2, 92.4)
  line L7 (-172.2, 82.4) -> (-202.2, 82.4)
  line L8 (-202.2, 82.4) -> (-202.2, 92.4)
  line L9 (-350, 92.4) -> (-187.2, 92.4)
  line L10 (-207.2, 101.8) -> (-207.2, 92.4)
  line L11 (-172.2, 92.4) -> (-172.2, 82.4)
  line L12 (-187.2, 81.8) -> (-187.2, 92.4)
  line L13 (-172.2, 82.4) -> (-162.2, 82.4)
  line L14 (-162.2, 82.4) -> (-162.2, 92.4)
  line L15 (-162.2, 92.4) -> (-172.2, 92.4)
  line L16 (-172.2, 92.4) -> (-172.2, 82.4)
  line L17 (-92.2, 92.4) -> (-187.2, 92.4)
  circle A1 centre (-179.7, 87.4) radius 1.25
  dimension "d452" = 30
  dimension "d453" = 10
  dimension "d463" = 15
  dimension "d464" = 10
  dimension "d480" = 2.5
  dimension "d481" = 7.5
  dimension "d482" = 5
  constraint horizontal L6
  constraint horizontal L7
  constraint vertical L8
  constraint coincident L6.start L9
  constraint vertical L11
  constraint vertical L12
  constraint coincident L9.end L12.end
  constraint horizontal L13
  constraint vertical L14
  constraint horizontal L15
  constraint vertical L16
  constraint coincident L14.end L17
  measures "d452" distance of L6.start L6.end
  measures "d453" distance of L6.start L7.end
  measures "d463" distance of L2.end L8
  measures "d464" distance of L7.start L13.end
  measures "d480" diameter of A1
  measures "d481" distance of L11 A1.centre
  measures "d482" distance of L6 A1.centre
extrude "Extrusion38" add sketch "Skizze23" along normal blind 2.4 separate body contours L6 L7 L8 L9 L12 | L6 L7 L11 L12 L16 L17 | A1 makes body 22
extrude "Extrusion40" add sketch "Skizze23" along normal blind 4.8 separate body contours L11 L13 L14 L15 L16 L17 makes body 23
extrude "Extrusion41" add sketch "Skizze23" along normal blind 2.4 from surface at 2.4 separate body contours L6 L7 L11 L12 L16 L17 | A1 makes body 24
extrude "Extrusion42" add sketch "Skizze23" against normal blind 2.4 from surface at 129 separate body contours L6 L7 L8 L9 L12 | L6 L7 L11 L12 L16 L17 | A1 makes body 25
extrude "Extrusion43" add sketch "Skizze23" against normal blind 4.8 from surface at 129 separate body contours L11 L13 L14 L15 L16 L17 makes body 26
extrude "Extrusion44" add sketch "Skizze23" against normal blind 2.4 from surface at 126.6 separate body contours L6 L7 L11 L12 L16 L17 | A1 makes body 27
combine "Kombinieren4" operation add target body 12 tool bodies 22 25
combine "Kombinieren5" operation add target body 16 tool bodies 26 27 24 23
extrude "Extrusion45" cut sketch "Skizze23" along normal up to surface (133.8 mm away) from surface at -2.4 contours A1 bodies 12 16
split "Teilen2" by curves path "Skizze21" along L29 bodies 3 makes body 28 at (69.8, 99.4, 282.8333)
chamfer "Fase3" distance 7 distance2 9.4 3 edges at (-8.2, 101.8, 72.2) (-8.2, 101.8, 305) (-8.2, 101.8, 187.2) measured on face at (-7.8, 101.8, 85.5333) measured on face at (-7.8, 101.8, 311.6667) measured on face at (-7.8, 101.8, 193.8667) on bodies 12 16
chamfer "Fase4" distance 9.4 distance2 7 3 edges at (-8.2, 101.8, 92.2) (-8.2, 101.8, 325) (-8.2, 101.8, 207.2) measured on face at (-7.8, 95.5333, 92.2) measured on face at (-8.6, 98.6667, 325) measured on face at (-8.6, 95.5333, 207.2) on bodies 12 16